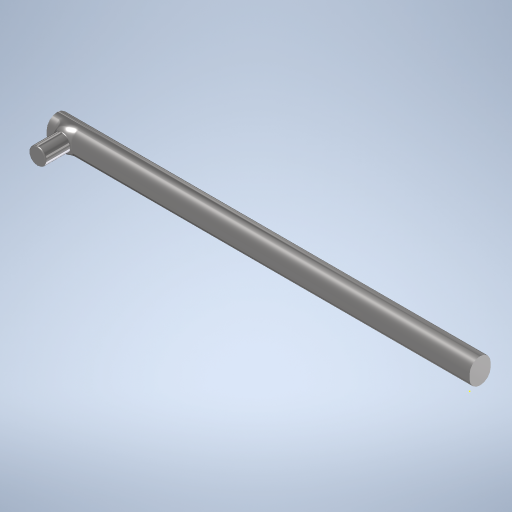
# Autodesk Inventor part: clamp_rod
Saved by Autodesk Inventor 2023 (Build 270158000, 158)
## iProperties
Created: 2023-11-21
Part Number: clamp_rod
Material: Steel, Mild
Document SubType Name: Modeling
Designer: Beatrice
Density: 7.85 g/cm^3
Appearance: Semi-Polished
Author: Beatrice
Autodesk Inventor part; units mm, degrees
ref_plane "YZ Plane" through (0, 0, 0) normal (1, 0, 0) x (0, 1, 0)
ref_plane "XZ Plane" through (0, 0, 0) normal (0, 1, 0) x (-1, 0, 0)
ref_plane "XY Plane" through (0, 0, 0) normal (0, 0, 1) x (1, 0, 0)
sketch "Sketch1" plane through (0, 0, 0) normal (1, 0, 0) x (0, 1, 0)
  line L0 (0, 0) -> (1, 0)
  line L1 (1, 0) -> (1, 1.2)
  line L2 (1, 1.2) -> (0, 1.2)
  line L3 (0, 1.2) -> (0, 0)
  dimension "d0" = 1
  dimension "d1" = 1.2
  constraints: 8 end point, 2 parallel, 1 horizontal, 1 perpendicular
  measures "d0" distance of L2.end L1.end
  measures "d1" distance of L1.end L0.end
extrude "Extrusion1" add sketch "Sketch1" along normal blind 20
sketch "Sketch2" plane through (0, 0, 0) normal (0, -1, 0) x (1, 0, 0)
  line L0 (0, 0) -> (0, 1.2) projected
  line L1 (0, 0.6) -> (4, 0.6) construction
  circle A0 centre (0.75, 0.6) radius 0.4
  line L2 (20, 1.2) -> (20, 0) projected
  dimension "d4" = 0.8
  dimension "d5" = 19.25
  constraints: 2 end point, 1 centre point, 1 horizontal, 1 midpoint, 1 point on line
  measures "d4" diameter of A0
  measures "d5" distance from line of L2 A0.centre
extrude "Extrusion2" add sketch "Sketch2" along normal blind 1.2
fillet "Fillet2" radius 0.06 2 edges at (0.35, 0, 0.6) (0.35, -1.2, 0.6)
fillet "Fillet3" radius 0.5 4 edges at (10, 1, 0) (10, 1, 1.2) (10, 0, 1.2) (10, 0, 0)
sketch "Sketch3" plane through (20, 0, 0) normal (1, 0, 0) x (0, 0, -1)
  point P0 (0, 0)
body "Solid1"
